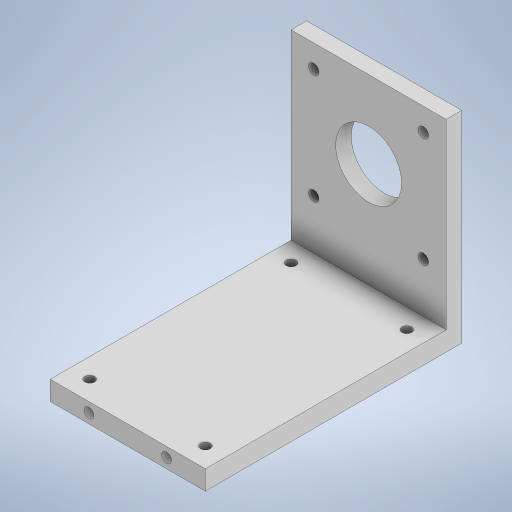
# Autodesk Inventor part: FloorMount
Saved by Autodesk Inventor 2024 (Build 280153000, 153)
## iProperties
Created: 2024-02-13
Part Number: FloorMount
Material: Generic
Document SubType Name: Modeling
Designer: yusuf
Density: 1 g/cm^3
Appearance: Default
Author: yusuf
Autodesk Inventor part; units mm, degrees
ref_plane "YZ Plane" through (0, 0, 0) normal (1, 0, 0) x (0, 1, 0)
ref_plane "XZ Plane" through (0, 0, 0) normal (0, 1, 0) x (-1, 0, 0)
ref_plane "XY Plane" through (0, 0, 0) normal (0, 0, 1) x (1, 0, 0)
sketch "Sketch1" plane through (0, 0, 0) normal (0, 0, 1) x (1, 0, 0)
  line L0 (0, 0) -> (200, 0)
  line L1 (200, 0) -> (200, 260)
  line L2 (200, 260) -> (0, 260)
  line L3 (0, 260) -> (0, 0)
  dimension "d0" = 200
  dimension "d1" = 260
  constraints: 8 end point, 2 parallel, 1 horizontal, 1 perpendicular
  measures "d0" distance of L1.end L2.end
  measures "d1" distance of L0.end L1.end
extrude "Extrusion1" add sketch "Sketch1" along normal blind 20
sketch "Sketch2" plane through (0, 0, 20) normal (0, 0, 1) x (1, 0, 0)
  circle A0 centre (100, 160) radius 42.5
  line L0 (200, 260) -> (0, 260) projected
  line L1 (0, 260) -> (0, 0) projected
  dimension "d4" = 85
  dimension "d5" = 100
  dimension "d6" = 100
  constraints: 1 centre point
  measures "d4" diameter of A0
  measures "d5" distance from line of A0.centre L0
  measures "d6" distance from line of L1 A0.centre
extrude "Extrusion2" cut sketch "Sketch2" against normal blind 30
sketch "Sketch3" plane through (0, 0, 20) normal (0, 0, 1) x (1, 0, 0)
  line L0 (0, 260) -> (0, 0) projected
  line L1 (200, 0) -> (200, 260) projected
  line L2 (0, 0) -> (200, 0)
  line L3 (200, 0) -> (200, 25)
  line L4 (200, 25) -> (0, 25)
  line L5 (0, 25) -> (0, 0)
  point P0 (0, 25)
  dimension "d9" = 25
  constraints: 8 end point, 2 parallel, 1 horizontal, 1 perpendicular, 1 point on line
  measures "d9" distance of L1.start L3.end
extrude "Extrusion3" add sketch "Sketch3" along normal blind 330.6
sketch "Sketch4" plane through (0, 25, 20) normal (0, 1, 0) x (1, 0, 0)
  line L0 (0, 20) -> (0, -330.6) projected
  line L1 (200, 20) -> (200, -330.6) projected
  line L2 (0, -330.6) -> (200, -330.6)
  line L3 (200, -330.6) -> (200, -310.6)
  line L4 (200, -310.6) -> (0, -310.6)
  line L5 (0, -310.6) -> (0, -330.6)
  point P0 (0, -310.6)
  dimension "d12" = 20
  constraints: 8 end point, 2 parallel, 1 horizontal, 1 perpendicular, 1 point on line
  measures "d12" distance of L3.end L1.end
extrude "Extrusion4" add sketch "Sketch4" along normal blind 350
sketch "Sketch5" plane through (200, 25, 330.6) normal (0, 0, -1) x (-1, 0, 0)
  circle A0 centre (100, 135) radius 42.5 projected
  circle A1 centre (100, 135) radius 42.5
  point P0 (200, -25)
  dimension "d15" = 85
  constraints: 1 centre point, 1 coincident
  measures "d15" diameter of A1
extrude "Extrusion5" cut sketch "Sketch5" against normal blind 20
sketch "Sketch6" plane through (0, 0, 0) normal (0, 0, -1) x (-1, 0, 0)
  circle A0 centre (-29.289, 230.711) radius 6.75
  circle A1 centre (-170.711, 230.711) radius 6.75
  circle A2 centre (-170.711, 89.289) radius 6.75
  circle A3 centre (-29.289, 89.289) radius 6.75
  circle A4 centre (-100, 160) radius 42.5 projected
  point P0 (0, 0)
  dimension "d18" = 70.711
  dimension "d19" = 70.711
  dimension "d20" = 70.711
  dimension "d21" = 70.711
  dimension "d22" = 70.711
  dimension "d23" = 70.711
  dimension "d24" = 70.711
  dimension "d25" = 70.711
  dimension "d26" = 13.5
  dimension "d27" = 13.5
  dimension "d28" = 13.5
  dimension "d29" = 13.5
  constraints: 4 centre point
  measures "d18" horizontal distance of A4.centre A2.centre
  measures "d19" horizontal distance of A4.centre A2.centre
  measures "d20" horizontal distance of A4.centre A1.centre
  measures "d21" horizontal distance of A4.centre A1.centre
  measures "d22" horizontal distance of A4.centre A0.centre
  measures "d23" horizontal distance of A4.centre A0.centre
  measures "d24" horizontal distance of A4.centre A3.centre
  measures "d25" horizontal distance of A4.centre A3.centre
  measures "d26" diameter of A1
  measures "d27" diameter of A0
  measures "d28" diameter of A3
  measures "d29" diameter of A2
extrude "Extrusion6" cut sketch "Sketch6" against normal blind 20 contours A0 | A1 | A2 | A3
sketch "Sketch7" plane through (200, 0, 0) normal (1, 0, 0) x (0, 0, -1)
  line L0 (-350.6, 0) -> (-350.6, 375) projected
  line L1 (0, 0) -> (-350.6, 0) projected
  line L2 (-350.6, 375) -> (-330.6, 375)
  line L3 (-330.6, 375) -> (-330.6, 0)
  line L4 (-330.6, 0) -> (-350.6, 0)
  line L5 (-350.6, 0) -> (-350.6, 375)
  dimension "d32" = 20
  constraints: 8 end point, 2 parallel, 1 horizontal, 1 perpendicular, 1 point on line
  measures "d32" distance of L3.end L0.start
extrude "Extrusion7" cut sketch "Sketch7" against normal blind 200
sketch "Sketch9" plane through (200, 0, 330.6) normal (0, 0, 1) x (1, 0, 0)
  circle A0 centre (-150, 12.5) radius 6.35
  circle A1 centre (-50, 12.5) radius 6.35
  line L0 (-200, 0) -> (-200, 25) projected
  line L1 (0, 25) -> (0, 0) projected
  line L2 (0, 0) -> (-200, 0) projected
  point P0 (-200, 12.5)
  dimension "d35" = 12.7
  dimension "d36" = 12.7
  dimension "d37" = 50
  dimension "d38" = 50
  dimension "d39" = 12.5
  dimension "d40" = 12.5
  constraints: 2 centre point, 1 midpoint
  measures "d35" diameter of A0
  measures "d36" diameter of A1
  measures "d37" distance of point (-200, 12.5) A0.centre
  measures "d38" distance from line of L1 A1.centre
  measures "d39" distance from line of L2 A1.centre
  measures "d40" distance from line of L2 A0.centre
extrude "Extrusion8" cut sketch "Sketch9" against normal blind 20
sketch "Sketch10" plane through (0, 25, 20) normal (0, 1, 0) x (1, 0, 0)
  circle A0 centre (25.4, -25.4) radius 6.35
  circle A1 centre (174.6, -25.4) radius 6.35
  circle A2 centre (25.4, -285.2) radius 6.35
  circle A3 centre (174.6, -285.2) radius 6.35
  line L0 (0, 0) -> (0, -310.6) projected
  line L1 (0, -310.6) -> (200, -310.6) projected
  line L2 (200, 0) -> (200, -310.6) projected
  line L3 (0, 0) -> (200, 0) projected
  point P0 (0, 20)
  dimension "d43" = 25.4
  dimension "d44" = 25.4
  dimension "d45" = 12.7
  dimension "d46" = 25.4
  dimension "d47" = 25.4
  dimension "d48" = 12.7
  dimension "d49" = 25.4
  dimension "d50" = 25.4
  dimension "d51" = 25.4
  dimension "d52" = 25.4
  dimension "d53" = 12.7
  dimension "d54" = 12.7
  constraints: 4 centre point
  measures "d43" distance from line of L0 A2.centre
  measures "d44" distance from line of L1 A2.centre
  measures "d45" diameter of A2
  measures "d46" distance from line of L2 A3.centre
  measures "d47" distance from line of L1 A3.centre
  measures "d48" diameter of A3
  measures "d49" distance from line of L2 A1.centre
  measures "d50" distance from line of L3 A1.centre
  measures "d51" distance from line of L3 A0.centre
  measures "d52" distance from line of L0 A0.centre
  measures "d53" diameter of A0
  measures "d54" diameter of A1
extrude "Extrusion9" cut sketch "Sketch10" against normal blind 25.4 contours A0 | A1 | A2 | A3
equation "\"d19\" = d18"
equation "\"d20\" = d18"
equation "\"d21\" = d19"
equation "\"d22\" = d20"
equation "\"d23\" = d22"
equation "\"d24\" = d23"
equation "\"d25\" = d23"
equation "\"d40\" = d39"
equation "\"d48\" = d45"
equation "\"d49\" = d46"
equation "\"d50\" = d49"
equation "\"d51\" = d50"
equation "\"d52\" = d51"
equation "\"d53\" = d48"
equation "\"d54\" = d53"
body "Solid1"
